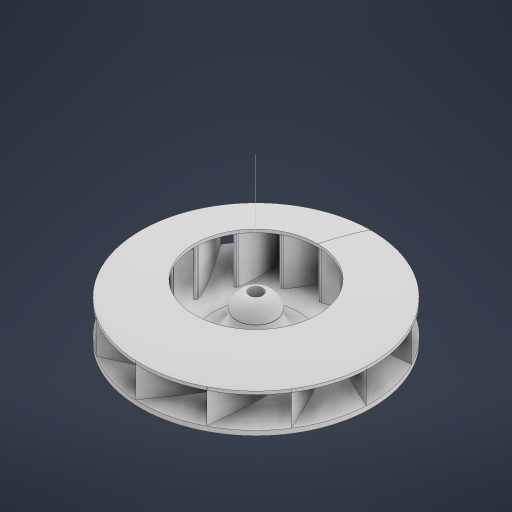
# Autodesk Inventor part: FanWing
Saved by Autodesk Inventor 2023 (Build 270158000, 158)
## iProperties
Created: 2023-02-14
Part Number: FanWing
Material: 一般
Document SubType Name: Modeling
Designer: neko2
Density: 1 g/cm^3
Appearance: 既定
Author: neko2
Autodesk Inventor part; units mm, degrees
ref_plane "YZ Plane" through (0, 0, 0) normal (1, 0, 0) x (0, 1, 0)
ref_plane "XZ Plane" through (0, 0, 0) normal (0, 1, 0) x (-1, 0, 0)
ref_plane "XY Plane" through (0, 0, 0) normal (0, 0, 1) x (1, 0, 0)
sketch "スケッチ1" plane through (0, 0, 0) normal (0, 1, 0) x (-1, 0, 0)
  circle A0 centre (0, 0) radius 7.5
  dimension "d0" = 15
  constraints: 1 centre point, 1 coincident
  measures "d0" diameter of A0
extrude "押し出し1" add sketch "スケッチ1" along normal blind 0.3
sketch "スケッチ2" plane through (0, 0.3, 0) normal (0, 1, 0) x (1, 0, 0)
  circle A0 centre (0, 0) radius 7.5 projected
  line L0 (-4, 0) -> (-6.326, 4.0288)
  line L1 (-4, 0) -> (-4.5, 0) construction
  line L2 (-4.5, 0) -> (-6.326, 4.0288) construction
  spline S0 degree 2 poles (-4, 0) (-4.5, 0) (-6.326, 4.0288) knots 1 1 1 2 2 2
  line L3 (-4, 0) -> (-4, 2.578)
  line L4 (0, 0) -> (-7.5, 0)
  line L5 (-4, 0) -> (-3.75, 0.433) construction
  line L6 (-3.75, 0.433) -> (-6.326, 4.0288) construction
  spline S1 degree 2 poles (-4, 0) (-3.75, 0.433) (-6.326, 4.0288) knots 1 1 1 2 2 2
  point P0 (-4, 0.2522)
  dimension "d22" = 30
  dimension "d24" = 0.5
  dimension "d25" = 4
  constraints: 6 end point, 2 point on circle, 2 point on line, 1 horizontal, 1 symmetric about line, 1 vertical, 6 other
  measures "d22" angle of L3 L0
  measures "d24" distance of L0.start L1.end
  measures "d25" distance of point (0, 0) L0.start
extrude "押し出し2" add sketch "スケッチ2" along normal blind 3 contours S1 L3 L0 | L0 S0 | L3 S1
fillet "フィレット1" radius 0.1 1 edges at (-4, 1.8, 0)
pattern_circular "円形状パターン1" count 12 over 360 about axis through (0, 0, 0) along (0, 1, 0) of "押し出し2", "フィレット1"
sketch "スケッチ3" plane through (0, 0.3, 0) normal (0, 1, 0) x (1, 0, 0)
  circle A0 centre (0, 0) radius 1.25
  dimension "d17" = 2.5
  constraints: 1 centre point, 1 coincident
  measures "d17" diameter of A0
extrude "押し出し3" add sketch "スケッチ3" along normal blind 2.5
fillet "フィレット3" radius 1.5 1 edges at (-1.25, 0.3, 0)
sketch "スケッチ4" plane through (0, 2.8, 0) normal (0, 1, 0) x (1, 0, 0)
  circle A0 centre (0, 0) radius 0.425
  dimension "d21" = 0.85
  constraints: 1 centre point, 1 coincident
  measures "d21" diameter of A0
extrude "押し出し4" cut sketch "スケッチ4" against normal through all
sketch "スケッチ6" plane through (0, 0, 0) normal (1, 0, 0) x (0, 1, 0)
  line L0 (0, -7.5) -> (0, 7.5) projected
  line L1 (0, -7.5) -> (0.3, -7.5)
  line L2 (0, -7.5) -> (0.3, -7.5) projected
  line L3 (0.3, -7.5) -> (0.3, -6.6521) projected
  line L4 (0.3, -7.4929) -> (3.3, -7.4929) projected
  line L5 (3.5, -4) -> (3.3, -4)
  line L6 (3.3, -4) -> (2.6, -7) construction
  line L7 (2.6, -7) -> (2.3, -7.5) construction
  spline S0 degree 2 poles (3.3, -4) (2.6, -7) (2.3, -7.5) knots 1 1 1 2 2 2
  line L8 (3.5, -4) -> (2.8, -7) construction
  line L9 (2.8, -7) -> (2.5, -7.5) construction
  spline S1 degree 2 poles (3.5, -4) (2.8, -7) (2.5, -7.5) knots 1 1 1 2 2 2
  line L10 (2.5, -7.5) -> (2.3, -7.5)
  line L11 (2.8, -7) -> (2.6, -7)
  line L12 (-0.7554, 0) -> (4.5322, 0) projected
  line L13 (3.3, -7.4929) -> (3.5, -4)
  line L14 (3.3, -7.4929) -> (3.3, -7.9929)
  line L15 (3.3, -7.9929) -> (2.3, -7.9929)
  line L16 (2.3, -7.9929) -> (2.3, -7.5)
  point P0 (0, 0)
  point P1 (3.4, -4)
  point P2 (2.3042, -7.4929)
  point P3 (2.5042, -7.4929)
  dimension "d26" = 0.2
  dimension "d28" = 4
  dimension "d29" = 2
  dimension "d30" = 3
  dimension "d31" = 0.5
  dimension "d32" = 0.3
  dimension "d35" = 0.5
  constraints: 16 end point, 3 parallel, 2 coincident, 2 horizontal, 2 horizontal alignment, 2 perpendicular, 1 midpoint, 1 point on line, 1 vertical, 6 other
  measures "d26" distance of L5.start L5.end
  measures "d28" distance from line of point (3.4, -4) L12
  measures "d29" distance of L4.start L7.end
  measures "d30" vertical distance of L5.end L6.end
  measures "d31" horizontal distance of L5.end L11.start
  measures "d32" horizontal distance of L7.end L6.end
  measures "d35" distance between parallel lines of L15 L4
fillet "フィレット4" radius 1 1 edges at (-1.25, 2.8, 0)
revolve "回転4" cut sketch "スケッチ6" angle 360 about axis through (0, 0, 0) along (0, 1, 0) contours S0 L5 S1 L4 | S1 L13 L4 | L4 L14 L15 L16 L10 S1
revolve "回転5" add sketch "スケッチ6" angle 360 about axis through (0, 0, 0) along (0, 1, 0) contours S0 L5 S1 L4
